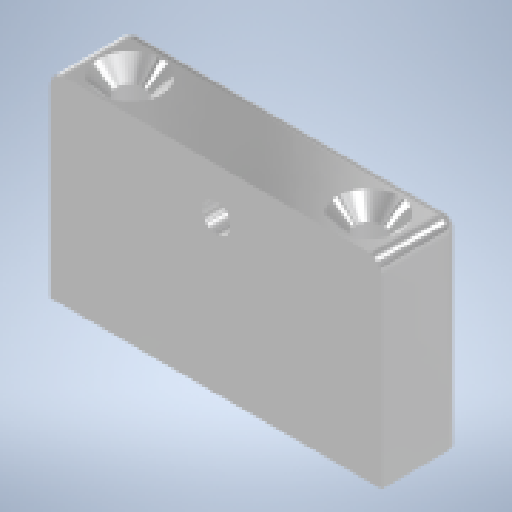
# Autodesk Inventor part: HebelhalterBlock
Saved by Autodesk Inventor 2025 (Build 290162010, 162A)
## iProperties
Created: 2024-11-27
Part Number: HebelhalterBlock
Material: Aluminium 6061(1)
Document SubType Name: Modeling
Designer: Admin
Density: 2.7 g/cm^3
Appearance: Aluminium - flach(1)
Author: Admin
Autodesk Inventor part; units mm, degrees
ref_plane "YZ Plane" through (0, 0, 0) normal (1, 0, 0) x (0, 1, 0)
ref_plane "XZ Plane" through (0, 0, 0) normal (0, 1, 0) x (-1, 0, 0)
ref_plane "XY Plane" through (0, 0, 0) normal (0, 0, 1) x (1, 0, 0)
sketch "Skizze1" plane through (0, 0, 0) normal (0, 0, 1) x (1, 0, 0)
  line L0 (140.5121, 9.5998) -> (90.5121, 9.5998)
  line L1 (90.5121, 9.5998) -> (90.5121, 21.5998)
  line L2 (90.5121, 21.5998) -> (140.5121, 21.5998)
  line L3 (140.5121, 21.5998) -> (140.5121, 9.5998)
  point P0 (0, 0)
  dimension "d0" = 50
  dimension "d1" = 12
  constraints: 8 end point, 2 parallel, 1 horizontal, 1 perpendicular
  measures "d0" distance of L1.end L2.end
  measures "d1" distance of L0.end L1.end
extrude "Extrusion1" add sketch "Skizze1" along normal blind 30
sketch "Skizze2" plane through (0, 0, 30) normal (0, 0, 1) x (1, 0, 0)
  line L0 (140.5121, 9.5998) -> (140.5121, 21.5998) projected
  line L1 (140.5121, 14.5998) -> (133.5121, 14.5998)
  line L2 (133.5121, 14.5998) -> (97.5121, 14.5998)
  line L3 (97.5121, 14.5998) -> (90.5121, 14.5998)
  line L4 (90.5121, 21.5998) -> (90.5121, 9.5998) projected
  line L5 (140.5121, 21.5998) -> (90.5121, 21.5998) projected
  point P0 (0, 0)
  dimension "d4" = 7
  dimension "d12" = 7
  constraints: 6 end point, 3 point on line, 2 coincident, 1 collinear, 1 horizontal, 1 perpendicular
  measures "d4" distance from line of L0 L1.end
  measures "d12" distance from line of L5 L1.start
hole "Bohrung1" at (133.5121, 14.5998, 30) at (97.5121, 14.5998, 30) direction (0, 0, -1) diameter 4.3 end through all countersink diameter 9.4 countersink angle 90 clearance for "Flachkopfmaschinenschraube" size "M4" standard "ANSI Metrisches M Profil"
sketch "Skizze4" plane through (90.5121, 21.5998, 0) normal (0, 1, 0) x (1, 0, 0)
  line L0 (25, -23) -> (25, -30)
  line L1 (50, -30) -> (0, -30) projected
  point P0 (-90.5121, 0)
  dimension "d37" = 7
  constraints: 2 end point, 1 midpoint, 1 perpendicular
  measures "d37" distance of L0.start L0.end
hole "Bohrung5" at (115.5121, 21.5998, 23) direction (0, -1, 0) diameter 4.3 end through all countersink diameter 9.4 countersink angle 90 clearance for "Flachkopfmaschinenschraube" size "M4" standard "ANSI Metrisches M Profil"
fillet "Rundung3" radius 2 5 edges at (140.5121, 15.5998, 30) (140.5121, 21.5998, 15) (115.5121, 21.5998, 30) (90.5121, 21.5998, 15) (90.5121, 15.5998, 30)
